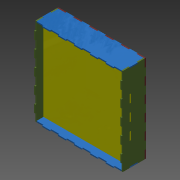
# Autodesk Inventor part: wordClock
Saved by Autodesk Inventor 2015 (Build 190159000, 159)
## iProperties
Created: 2015-02-10
Part Number: wordClock
Material: Generic
Document SubType Name: Modeling
Designer: Iain
Density: 1 g/cm^3
Appearance: Default
Author: Iain
Autodesk Inventor part; units mm, degrees
ref_plane "YZ Plane" through (0, 0, 0) normal (1, 0, 0) x (0, 1, 0)
ref_plane "XZ Plane" through (0, 0, 0) normal (0, 1, 0) x (-1, 0, 0)
ref_plane "XY Plane" through (0, 0, 0) normal (0, 0, 1) x (1, 0, 0)
sketch "Sketch1" plane through (0, 0, 0) normal (0, 0, 1) x (1, 0, 0)
  line L0 (-105, 105) -> (105, 105)
  line L1 (105, 105) -> (105, -105)
  line L2 (105, -105) -> (-105, -105)
  line L3 (-105, -105) -> (-105, 105)
  point P0 (0, 0)
  point P1 (0, 105)
  point P2 (-105, 0)
  dimension "FrontFaceBaseWidth" = 210
  dimension "FrontFaceBaseHeight" = 210
  constraints: 8 end point, 2 midpoint, 2 parallel, 1 horizontal, 1 horizontal alignment, 1 perpendicular, 1 vertical alignment
  measures "FrontFaceBaseWidth" distance of L0.start L0.end
  measures "FrontFaceBaseHeight" distance of L2.end L0.start
extrude "FrontFaceBase" add sketch "Sketch1" along normal mid plane 3
sketch "Sketch4" plane through (0, 0, 1.5) normal (0, 0, 1) x (1, 0, 0)
  line L0 (-108, 108) -> (-88, 108)
  line L1 (-88, 108) -> (-88, 105)
  line L2 (-88, 105) -> (-108, 105)
  line L3 (-108, 105) -> (-108, 108)
  point P0 (-105, 105)
  point P1 (0, 0)
  point P2 (-98, 105)
  dimension "d6" = 3
  dimension "FrontFaceTabWidth" = 20
  dimension "d8" = 3
  constraints: 8 end point, 2 parallel, 1 horizontal, 1 horizontal alignment, 1 midpoint, 1 perpendicular
  measures "d6" distance of point (-105, 105) L2.end
  measures "FrontFaceTabWidth" distance of L0.end L0.start
  measures "d8" distance of L1.end L0.end
extrude "Extrusion2" add sketch "Sketch4" against normal blind 3
pattern_linear "FrontTopTabs" count 6 spacing 39.2 along (1, 0, 0) of "Extrusion2"
sketch "Sketch5" plane through (0, 0, 1.5) normal (0, 0, 1) x (1, 0, 0)
  line L0 (-108, -108) -> (-105, -108)
  line L1 (-105, -108) -> (-105, -88)
  line L2 (-105, -88) -> (-108, -88)
  line L3 (-108, -88) -> (-108, -108)
  point P0 (-105, -105)
  point P1 (0, 0)
  point P2 (-105, -98)
  dimension "d14" = 3
  dimension "d15" = 3
  dimension "d16" = 20
  constraints: 8 end point, 2 parallel, 1 horizontal, 1 midpoint, 1 perpendicular, 1 vertical alignment
  measures "d14" distance of point (-105, -105) L0.end
  measures "d15" distance of L0.start L0.end
  measures "d16" distance of L2.end L0.start
extrude "Extrusion3" add sketch "Sketch5" against normal blind 3
pattern_linear "FontLeftTabs" count 6 spacing 39.2 along (0, 1, 0) of "Extrusion3"
mirror "FrontBottomTabs" about plane through (0, 0, 0) normal (0, 1, 0) of "Extrusion2", "FrontTopTabs"
mirror "FontRightTabs" about plane through (0, 0, 0) normal (1, 0, 0) of "Extrusion3", "FontLeftTabs"
sketch "Sketch6" plane through (-9.6, 105, -1.5) normal (0, 1, 0) x (1, 0, 0)
  line L0 (-98.4, -3) -> (117.6, -3)
  line L1 (117.6, -3) -> (117.6, 57)
  line L2 (117.6, 57) -> (-98.4, 57)
  line L3 (-98.4, 57) -> (-98.4, -3)
  line L4 (-59.2, -3) -> (-78.4, -3) projected
  line L5 (-98.4, -3) -> (-98.4, 0) projected
  point P0 (117.6, 27)
  point P1 (9.6, -3)
  point P2 (-68.8, -3)
  point P3 (-98.4, 27)
  point P4 (-98.4, -1.5)
  dimension "d68" = 216
  dimension "d69" = 60
  constraints: 8 end point, 5 midpoint, 2 parallel, 1 horizontal, 1 horizontal alignment, 1 perpendicular, 1 vertical alignment
  measures "d68" distance of L0.start L0.end
  measures "d69" distance of L0.end L1.end
extrude "TopFaceBase" add sketch "Sketch6" along normal blind 3 separate body
sketch "Sketch7" plane through (-9.6, 108, -1.5) normal (0, 1, 0) x (1, 0, 0)
  line L0 (-98.4, -3) -> (117.6, -3) projected
  line L1 (-98.4, 57) -> (-98.4, -3) projected
  line L2 (-98.4, -3) -> (-78.4, -3)
  line L3 (-78.4, -3) -> (-78.4, 0)
  line L4 (-78.4, 0) -> (-98.4, 0)
  line L5 (-98.4, 0) -> (-98.4, -3)
  point P0 (9.6, -1.5)
  point P1 (-98.4, 27)
  point P2 (9.6, -3)
  dimension "d25" = 20
  dimension "TopFaceFrontSlotDepth" = 3
  constraints: 8 end point, 2 midpoint, 2 parallel, 1 horizontal, 1 horizontal alignment, 1 perpendicular, 1 vertical alignment
  measures "d25" distance of L3.end L4.end
  measures "TopFaceFrontSlotDepth" distance of L2.start L4.end
extrude "Extrusion5" cut sketch "Sketch7" against normal blind 3 bodies 2
sketch "Sketch8" plane through (-9.6, 108, -1.5) normal (0, 1, 0) x (1, 0, 0)
  line L0 (117.6, -3) -> (114.6, -3)
  line L1 (114.6, -3) -> (114.6, 17)
  line L2 (114.6, 17) -> (117.6, 17)
  line L3 (117.6, 17) -> (117.6, -3)
  point P0 (9.6, -1.5)
  dimension "TopSideSlotWidth" = 20
  dimension "d33" = 3
  constraints: 8 end point, 2 parallel, 1 horizontal, 1 perpendicular
  measures "TopSideSlotWidth" distance of L0.end L1.end
  measures "d33" distance of L0.start L0.end
extrude "Extrusion6" cut sketch "Sketch8" against normal blind 3 bodies 2
pattern_linear "TopFrontSlots" count 6 spacing 39.2 along (1, 0, 0) of "Extrusion5", "Extrusion2" bodies 2
pattern_linear "TopSideRightSlots" count 2 spacing 40 along (0, 0, -1) of "Extrusion6" bodies 2
ref_plane "Work Plane1" through (-48.8, 108, -28.5) normal (0, 0, 1) x (1, 0, 0)
mirror "TopBackSlots" about plane through (-48.8, 108, -28.5) normal (0, 0, 1) of "Extrusion5", "Extrusion2", "TopFrontSlots" bodies 2
ref_plane "Work Plane2" through (0, 105, -18.5) normal (1, 0, 0) x (0, 0, -1)
mirror "TopSideLeftSlots" about plane through (0, 105, -18.5) normal (1, 0, 0) of "Extrusion6", "TopSideRightSlots" bodies 2
sketch "Sketch12" plane through (108, 105, -18.5) normal (1, 0, 0) x (0, 0, -1)
  line L0 (0, 0) -> (20, 0) projected
  line L1 (-20, 0) -> (40, 0)
  line L2 (40, 0) -> (40, -210)
  line L3 (40, -210) -> (-20, -210)
  line L4 (-20, -210) -> (-20, 0)
  line L5 (-17, -95.4) -> (-17, -114.6) projected
  line L6 (-20, -114.6) -> (-20, -95.4) projected
  point P0 (-18.5, -105)
  point P1 (10, 0)
  point P2 (10, 0)
  point P3 (-20, -105)
  point P4 (-17, -105)
  point P5 (-20, -105)
  dimension "SideFaceBaseHeight" = 210
  dimension "SideFaceBaseDepth" = 60
  constraints: 8 end point, 5 midpoint, 2 coincident, 2 parallel, 1 horizontal, 1 perpendicular
  measures "SideFaceBaseHeight" distance of L3.end L1.start
  measures "SideFaceBaseDepth" distance of L1.start L1.end
extrude "RightFaceBase" add sketch "Sketch12" against normal blind 3 separate body
sketch "Sketch13" plane through (108, 105, -18.5) normal (1, 0, 0) x (0, 0, -1)
  line L0 (-20, 0) -> (40, 0) projected
  line L1 (-20, 3) -> (0, 3)
  line L2 (0, 3) -> (0, 0)
  line L3 (0, 0) -> (-20, 0)
  line L4 (-20, 0) -> (-20, 3)
  line L5 (-20, -114.6) -> (-20, -95.4) projected
  point P0 (-18.5, -105)
  point P1 (-10, 0)
  point P2 (10, 0)
  point P3 (-20, 1.5)
  point P4 (-20, -105)
  dimension "SideFaceTabWidth" = 20
  dimension "SideTopTabDepth" = 3
  constraints: 8 end point, 4 midpoint, 2 parallel, 1 horizontal, 1 horizontal alignment, 1 perpendicular, 1 vertical alignment
  measures "SideFaceTabWidth" distance of L1.start L1.end
  measures "SideTopTabDepth" distance of L3.end L1.start
extrude "Extrusion9" add sketch "Sketch13" against normal blind 3 bodies 3
pattern_linear "SideTopTabs" count 2 spacing 40 along (0, 0, -1) of "Extrusion9" bodies 3
mirror "SideBottomTabs" about plane through (0, 0, 0) normal (0, 1, 0) of "Extrusion9", "SideTopTabs" bodies 3
sketch "Sketch14" plane through (108, 105, -18.5) normal (1, 0, 0) x (0, 0, -1)
  line L0 (-20, 3) -> (-20, -213) projected
  line L1 (-20, 3) -> (0, 3) projected
  line L2 (-20, 3) -> (-17, 3)
  line L3 (-17, 3) -> (-17, -17)
  line L4 (-17, -17) -> (-20, -17)
  line L5 (-20, -17) -> (-20, 3)
  point P0 (-18.5, -105)
  point P1 (-18.5, 3)
  point P2 (-10, 3)
  point P3 (-20, -7)
  point P4 (-20, -105)
  dimension "d61" = 3
  dimension "d62" = 20
  constraints: 8 end point, 4 midpoint, 2 parallel, 1 horizontal, 1 horizontal alignment, 1 perpendicular, 1 vertical alignment
  measures "d61" distance of L2.start L2.end
  measures "d62" distance of L4.end L2.start
extrude "Extrusion10" cut sketch "Sketch14" against normal blind 3 bodies 3
pattern_linear "SideFrontSlots" count 6 spacing 39.2 along (0, -1, 0) of "Extrusion10" bodies 3
ref_plane "Work Plane4" through (105, 29.6, -28.5) normal (0, 0, 1) x (1, 0, 0)
mirror "SideBackSlots" about plane through (105, 29.6, -28.5) normal (0, 0, 1) of "Extrusion10", "SideFrontSlots" bodies 3
mirror "Back" about plane through (105, 29.6, -28.5) normal (0, 0, 1) bodies 1 separate body
mirror "Left" about plane through (0, 105, -18.5) normal (1, 0, 0) bodies 3 separate body
mirror "Bottom" about plane through (0, 0, 0) normal (0, 1, 0) bodies 2 separate body
ref_plane "MiddleFacePlane" through (0, 0, -18.5) normal (0, 0, 1) x (1, 0, 0)
sketch "Sketch17" plane through (0, 0, -18.5) normal (0, 0, 1) x (1, 0, 0)
  line L0 (-105, 105) -> (105, 105)
  line L1 (105, 105) -> (105, -105)
  line L2 (105, -105) -> (-105, -105)
  line L3 (-105, -105) -> (-105, 105)
  point P0 (0, 0)
  point P1 (0, 105)
  point P2 (105, 0)
  dimension "d76" = 210
  dimension "d77" = 210
  constraints: 8 end point, 2 midpoint, 2 parallel, 1 horizontal, 1 horizontal alignment, 1 perpendicular, 1 vertical alignment
  measures "d76" distance of L0.end L1.end
  measures "d77" distance of L0.start L0.end
extrude "Extrusion13" add sketch "Sketch17" against normal blind 3 separate body
sketch "Sketch18" plane through (0, 0, -18.5) normal (0, 0, 1) x (1, 0, 0)
  line L0 (-105, -105) -> (-105, 105) projected
  line L1 (-105, -10) -> (-108, -10)
  line L2 (-108, -10) -> (-108, 10)
  line L3 (-108, 10) -> (-105, 10)
  line L4 (-105, 10) -> (-105, -10)
  point P0 (0, 0)
  point P1 (-105, 0)
  point P2 (-105, 0)
  point P3 (-108, 0)
  dimension "d80" = 3
  dimension "MiddleTabWidth" = 20
  constraints: 8 end point, 3 midpoint, 2 parallel, 1 coincident, 1 horizontal, 1 horizontal alignment, 1 perpendicular
  measures "d80" distance of L2.end L3.end
  measures "MiddleTabWidth" distance of L1.end L2.end
extrude "Extrusion14" add sketch "Sketch18" against normal blind 3 bodies 7
pattern_linear "LeftMiddleTabs" count 3 spacing 40 along (0, 1, 0) of "Extrusion14" first direction both ways yes bodies 7
mirror "RightMiddleTabs" about plane through (0, 0, 0) normal (1, 0, 0) of "Extrusion14", "LeftMiddleTabs" bodies 7
sketch "Sketch19" plane through (0, 0, -18.5) normal (0, 0, 1) x (1, 0, 0)
  line L0 (105, -105) -> (-105, -105) projected
  line L1 (-10, -105) -> (10, -105)
  line L2 (10, -105) -> (10, -108)
  line L3 (10, -108) -> (-10, -108)
  line L4 (-10, -108) -> (-10, -105)
  point P0 (0, 0)
  point P1 (0, -105)
  point P2 (0, -105)
  dimension "d87" = 3
  dimension "MiddleBottomTabWidth" = 20
  constraints: 8 end point, 2 midpoint, 2 parallel, 1 coincident, 1 horizontal, 1 perpendicular, 1 vertical alignment
  measures "d87" distance of L1.end L2.end
  measures "MiddleBottomTabWidth" distance of L1.start L1.end
extrude "Extrusion15" add sketch "Sketch19" against normal blind 3 bodies 7
pattern_linear "Rectangular Pattern9" count 3 spacing 40 along (-1, 0, 0) of "Extrusion15" first direction both ways yes bodies 7
sketch "Sketch21" plane through (0, 0, -18.5) normal (0, 0, 1) x (1, 0, 0)
  line L0 (10, -108) -> (-10, -108) projected
  line L1 (-10, -105) -> (10, -105)
  line L2 (10, -105) -> (10, -108)
  line L3 (10, -108) -> (-10, -108)
  line L4 (-10, -108) -> (-10, -105)
  point P0 (0, 0)
  point P1 (0, -105)
  point P2 (0, -108)
  point P3 (0, -108)
  dimension "d94" = 3
  dimension "d95" = 20
  constraints: 8 end point, 3 midpoint, 2 parallel, 1 coincident, 1 horizontal, 1 perpendicular, 1 vertical alignment
  measures "d94" distance of L1.end L2.end
  measures "d95" distance of L1.start L1.end
extrude "Extrusion16" cut sketch "Sketch21" against normal blind 3 bodies 6
pattern_linear "BottomMiddleSlots" count 3 spacing 40 along (-1, 0, 0) of "Extrusion16" first direction both ways yes bodies 6
sketch "Sketch22" plane through (0, 0, -18.5) normal (0, 0, 1) x (1, 0, 0)
  line L0 (-108, -10) -> (-108, 10) projected
  line L1 (-108, 10) -> (-105, 10)
  line L2 (-105, 10) -> (-105, -10)
  line L3 (-105, -10) -> (-108, -10)
  line L4 (-108, -10) -> (-108, 10)
  point P0 (0, 0)
  point P1 (-105, 0)
  point P2 (-108, 0)
  point P3 (-108, 0)
  dimension "d101" = 3
  dimension "d102" = 20
  constraints: 8 end point, 3 midpoint, 2 parallel, 1 coincident, 1 horizontal, 1 horizontal alignment, 1 perpendicular
  measures "d101" distance of L1.end L1.start
  measures "d102" distance of L3.end L1.start
extrude "Extrusion17" cut sketch "Sketch22" against normal blind 3 bodies 5
pattern_linear "LeftMiddleSlots" count 3 spacing 40 along (0, 1, 0) of "Extrusion14", "Extrusion17" first direction both ways yes bodies 5
mirror "RightMiddleSlots" about plane through (0, 0, 0) normal (1, 0, 0) of "LeftMiddleSlots", "Extrusion14", "Extrusion17" bodies 3
sketch "Sketch15" plane through (0, 0, 1.5) normal (0, 0, 1) x (1, 0, 0)
  line L0 (88, 108) -> (108, 108) projected
  line L1 (88, 105) -> (88, 108) projected
  line L2 (88, 105) -> (68.8, 105) projected
  line L3 (68.8, 108) -> (68.8, 105) projected
  line L4 (48.8, 108) -> (68.8, 108) projected
  line L5 (48.8, 105) -> (48.8, 108) projected
  line L6 (48.8, 105) -> (29.6, 105) projected
  line L7 (29.6, 108) -> (29.6, 105) projected
  line L8 (9.6, 108) -> (29.6, 108) projected
  line L9 (9.6, 105) -> (9.6, 108) projected
  line L10 (9.6, 105) -> (-9.6, 105) projected
  line L11 (-9.6, 108) -> (-9.6, 105) projected
  line L12 (-29.6, 108) -> (-9.6, 108) projected
  line L13 (-29.6, 105) -> (-29.6, 108) projected
  line L14 (-29.6, 105) -> (-48.8, 105) projected
  line L15 (-48.8, 108) -> (-48.8, 105) projected
  line L16 (-68.8, 108) -> (-48.8, 108) projected
  line L17 (-68.8, 105) -> (-68.8, 108) projected
  line L18 (-68.8, 105) -> (-88, 105) projected
  line L19 (-88, 108) -> (-88, 105) projected
  line L20 (-108, 108) -> (-88, 108) projected
  line L21 (-108, 108) -> (-108, 88) projected
  line L22 (-108, 88) -> (-105, 88) projected
  line L23 (-105, 88) -> (-105, 68.8) projected
  line L24 (-105, 68.8) -> (-108, 68.8) projected
  line L25 (-108, 68.8) -> (-108, 48.8) projected
  line L26 (-108, 48.8) -> (-105, 48.8) projected
  line L27 (-105, 48.8) -> (-105, 29.6) projected
  line L28 (-105, 29.6) -> (-108, 29.6) projected
  line L29 (-108, 29.6) -> (-108, 9.6) projected
  line L30 (-108, 9.6) -> (-105, 9.6) projected
  line L31 (-105, 9.6) -> (-105, -9.6) projected
  line L32 (-105, -9.6) -> (-108, -9.6) projected
  line L33 (-108, -9.6) -> (-108, -29.6) projected
  line L34 (-108, -29.6) -> (-105, -29.6) projected
  line L35 (-105, -29.6) -> (-105, -48.8) projected
  line L36 (-105, -48.8) -> (-108, -48.8) projected
  line L37 (-108, -48.8) -> (-108, -68.8) projected
  line L38 (-108, -68.8) -> (-105, -68.8) projected
  line L39 (-105, -68.8) -> (-105, -88) projected
  line L40 (-105, -88) -> (-108, -88) projected
  line L41 (-108, -88) -> (-108, -108) projected
  line L42 (-108, -108) -> (-88, -108) projected
  line L43 (-88, -108) -> (-88, -105) projected
  line L44 (-88, -105) -> (-68.8, -105) projected
  line L45 (-68.8, -105) -> (-68.8, -108) projected
  line L46 (-68.8, -108) -> (-48.8, -108) projected
  line L47 (-48.8, -108) -> (-48.8, -105) projected
  line L48 (-48.8, -105) -> (-29.6, -105) projected
  line L49 (-29.6, -105) -> (-29.6, -108) projected
  line L50 (-29.6, -108) -> (-9.6, -108) projected
  line L51 (-9.6, -108) -> (-9.6, -105) projected
  line L52 (-9.6, -105) -> (9.6, -105) projected
  line L53 (9.6, -105) -> (9.6, -108) projected
  line L54 (9.6, -108) -> (29.6, -108) projected
  line L55 (29.6, -108) -> (29.6, -105) projected
  line L56 (29.6, -105) -> (48.8, -105) projected
  line L57 (48.8, -105) -> (48.8, -108) projected
  line L58 (48.8, -108) -> (68.8, -108) projected
  line L59 (68.8, -108) -> (68.8, -105) projected
  line L60 (68.8, -105) -> (88, -105) projected
  line L61 (88, -105) -> (88, -108) projected
  line L62 (88, -108) -> (108, -108) projected
  line L63 (108, -108) -> (108, -88) projected
  line L64 (105, -88) -> (108, -88) projected
  line L65 (105, -88) -> (105, -68.8) projected
  line L66 (108, -68.8) -> (105, -68.8) projected
  line L67 (108, -48.8) -> (108, -68.8) projected
  line L68 (105, -48.8) -> (108, -48.8) projected
  line L69 (105, -48.8) -> (105, -29.6) projected
  line L70 (108, -29.6) -> (105, -29.6) projected
  line L71 (108, -9.6) -> (108, -29.6) projected
  line L72 (105, -9.6) -> (108, -9.6) projected
  line L73 (105, -9.6) -> (105, 9.6) projected
  line L74 (108, 9.6) -> (105, 9.6) projected
  line L75 (108, 29.6) -> (108, 9.6) projected
  line L76 (105, 29.6) -> (108, 29.6) projected
  line L77 (105, 29.6) -> (105, 48.8) projected
  line L78 (108, 48.8) -> (105, 48.8) projected
  line L79 (108, 68.8) -> (108, 48.8) projected
  line L80 (105, 68.8) -> (108, 68.8) projected
  line L81 (105, 68.8) -> (105, 88) projected
  line L82 (108, 88) -> (105, 88) projected
  line L83 (108, 108) -> (108, 88) projected
  line L84 (-87, 109) -> (-87, 104)
  line L85 (-87, 104) -> (-69.8, 104)
  line L86 (-69.8, 104) -> (-69.8, 109)
  line L87 (-69.8, 109) -> (-47.8, 109)
  line L88 (-47.8, 109) -> (-47.8, 104)
  line L89 (-47.8, 104) -> (-30.6, 104)
  line L90 (-30.6, 104) -> (-30.6, 109)
  line L91 (-30.6, 109) -> (-8.6, 109)
  line L92 (-8.6, 109) -> (-8.6, 104)
  line L93 (-8.6, 104) -> (8.6, 104)
  line L94 (8.6, 104) -> (8.6, 109)
  line L95 (8.6, 109) -> (30.6, 109)
  line L96 (30.6, 109) -> (30.6, 104)
  line L97 (30.6, 104) -> (47.8, 104)
  line L98 (47.8, 104) -> (47.8, 109)
  line L99 (47.8, 109) -> (69.8, 109)
  line L100 (69.8, 109) -> (69.8, 104)
  line L101 (69.8, 104) -> (87, 104)
  line L102 (87, 104) -> (87, 109)
  line L103 (87, 109) -> (109, 109)
  line L104 (109, 109) -> (109, 87)
  line L105 (109, 87) -> (104, 87)
  line L106 (104, 87) -> (104, 69.8)
  line L107 (104, 69.8) -> (109, 69.8)
  line L108 (109, 69.8) -> (109, 47.8)
  line L109 (109, 47.8) -> (104, 47.8)
  line L110 (104, 47.8) -> (104, 30.6)
  line L111 (104, 30.6) -> (109, 30.6)
  line L112 (109, 30.6) -> (109, 8.6)
  line L113 (109, 8.6) -> (104, 8.6)
  line L114 (104, 8.6) -> (104, -8.6)
  line L115 (104, -8.6) -> (109, -8.6)
  line L116 (109, -8.6) -> (109, -30.6)
  line L117 (109, -30.6) -> (104, -30.6)
  line L118 (104, -30.6) -> (104, -47.8)
  line L119 (104, -47.8) -> (109, -47.8)
  line L120 (109, -47.8) -> (109, -69.8)
  line L121 (109, -69.8) -> (104, -69.8)
  line L122 (104, -69.8) -> (104, -87)
  line L123 (104, -87) -> (109, -87)
  line L124 (109, -87) -> (109, -109)
  line L125 (109, -109) -> (87, -109)
  line L126 (87, -109) -> (87, -104)
  line L127 (87, -104) -> (69.8, -104)
  line L128 (69.8, -104) -> (69.8, -109)
  line L129 (69.8, -109) -> (47.8, -109)
  line L130 (47.8, -109) -> (47.8, -104)
  line L131 (47.8, -104) -> (30.6, -104)
  line L132 (30.6, -104) -> (30.6, -109)
  line L133 (30.6, -109) -> (8.6, -109)
  line L134 (8.6, -109) -> (8.6, -104)
  line L135 (8.6, -104) -> (-8.6, -104)
  line L136 (-8.6, -104) -> (-8.6, -109)
  line L137 (-8.6, -109) -> (-30.6, -109)
  line L138 (-30.6, -109) -> (-30.6, -104)
  line L139 (-30.6, -104) -> (-47.8, -104)
  line L140 (-47.8, -104) -> (-47.8, -109)
  line L141 (-47.8, -109) -> (-69.8, -109)
  line L142 (-69.8, -109) -> (-69.8, -104)
  line L143 (-69.8, -104) -> (-87, -104)
  line L144 (-87, -104) -> (-87, -109)
  line L145 (-87, -109) -> (-109, -109)
  line L146 (-109, -109) -> (-109, -87)
  line L147 (-109, -87) -> (-104, -87)
  line L148 (-104, -87) -> (-104, -69.8)
  line L149 (-104, -69.8) -> (-109, -69.8)
  line L150 (-109, -69.8) -> (-109, -47.8)
  line L151 (-109, -47.8) -> (-104, -47.8)
  line L152 (-104, -47.8) -> (-104, -30.6)
  line L153 (-104, -30.6) -> (-109, -30.6)
  line L154 (-109, -30.6) -> (-109, -8.6)
  line L155 (-109, -8.6) -> (-104, -8.6)
  line L156 (-104, -8.6) -> (-104, 8.6)
  line L157 (-104, 8.6) -> (-109, 8.6)
  line L158 (-109, 8.6) -> (-109, 30.6)
  line L159 (-109, 30.6) -> (-104, 30.6)
  line L160 (-104, 30.6) -> (-104, 47.8)
  line L161 (-104, 47.8) -> (-109, 47.8)
  line L162 (-109, 47.8) -> (-109, 69.8)
  line L163 (-109, 69.8) -> (-104, 69.8)
  line L164 (-104, 69.8) -> (-104, 87)
  line L165 (-104, 87) -> (-109, 87)
  line L166 (-109, 87) -> (-109, 109)
  line L167 (-109, 109) -> (-87, 109)
  point P0 (0, 0)
  dimension "d70" = 1
  constraints: 168 end point, 83 other
  measures "d70" distance between parallel lines of L20 L167
ref_plane "Work Plane3" through (0, 0, 0) normal (0, 1, 0) x (-1, 0, 0)
equation "\"FrontFaceBaseWidth\" = ClockWidth - 2 * FrontFaceTabDepth"
equation "\"FrontFaceBaseHeight\" = ClockHeight - 2 * FrontFaceTabDepth"
equation "\"FrontFaceThickness\" = Ply3mm"
equation "\"d6\" = TabDepth"
equation "\"FrontFaceTabWidth\" = TabWidth"
equation "\"d8\" = FrontFaceTabDepth"
equation "\"d9\" = FrontFaceThickness"
equation "\"d14\" = FrontFaceTabDepth"
equation "\"d15\" = FrontFaceTabDepth"
equation "\"d16\" = FrontFaceTabWidth"
equation "\"d17\" = FrontFaceThickness"
equation "\"d68\" = ClockWidth"
equation "\"d69\" = ClockDepth"
equation "\"TopFaceThickness\" = Ply3mm"
equation "\"d25\" = FrontFaceTabWidth"
equation "\"TopFaceFrontSlotDepth\" = FrontFaceThickness"
equation "\"d27\" = TopFaceThickness"
equation "\"d33\" = TabDepth"
equation "\"d34\" = TopFaceThickness"
equation "\"d38\" = FrontFaceTopTabSpacing"
equation "\"SideFaceBaseHeight\" = ClockHeight - 2 * FrontFaceThickness"
equation "\"SideFaceBaseDepth\" = ClockDepth"
equation "\"SideFaceThickness\" = Ply3mm"
equation "\"SideFaceTabWidth\" = TopSideSlotWidth"
equation "\"SideTopTabDepth\" = TopFaceThickness"
equation "\"d56\" = SideFaceThickness"
equation "\"d60\" = TopFaceSlotsSideSpcaing"
equation "\"d61\" = FrontFaceThickness"
equation "\"d62\" = FrontFaceTabWidth"
equation "\"d63\" = SideFaceThickness"
equation "\"d67\" = FrontFaceSideTabSpacing"
equation "\"d76\" = FrontFaceBaseHeight"
equation "\"d77\" = FrontFaceBaseWidth"
equation "\"MiddleThickness\" = Ply3mm"
equation "\"d80\" = SideFaceThickness"
equation "\"MiddleTabWidth\" = TabWidth"
equation "\"d82\" = Ply3mm"
equation "\"d86\" = MiddleSideTabSpacing"
equation "\"d87\" = TopFaceThickness"
equation "\"MiddleBottomTabWidth\" = MiddleTabWidth"
equation "\"d89\" = MiddleThickness"
equation "\"d93\" = MiddleBottomTabSpacing"
equation "\"d94\" = TopFaceThickness"
equation "\"d95\" = MiddleBottomTabWidth"
equation "\"d96\" = MiddleThickness"
equation "\"d100\" = MiddleBottomTabSpacing"
equation "\"d101\" = SideFaceThickness"
equation "\"d102\" = MiddleTabWidth"
equation "\"d103\" = MiddleThickness"
equation "\"d70\" = kerf"
equation "\"FrontFaceTabDepth\" = TabDepth"
equation "\"ClockHeight\" = 216"
equation "\"ClockWidth\" = 216"
equation "\"ClockDepth\" = 60"
equation "\"Ply3mm\" = 3"
equation "\"TabDepth\" = Ply3mm"
equation "\"TabWidth\" = 20"
equation "\"kerf\" = 1"
equation "\"MiddleFrontSeparation\" = 17"
equation "\"MiddleSideTabSpacing\" = 2 * MiddleTabWidth"
equation "\"MiddleBottomTabSpacing\" = MiddleSideTabSpacing"
equation "\"FrontFaceTopTabSpacing\" = 39.2"
equation "\"TopFaceSlotsSideSpcaing\" = 40"
equation "\"FrontFaceSideTabSpacing\" = 39.2"
